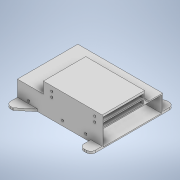
# Autodesk Inventor part: HardDriveHolder
Saved by Autodesk Inventor 2022 (Build 260153000, 153)
## iProperties
Created: 2021-08-26
Part Number: HardDriveHolder
Material: Generic
Document SubType Name: Modeling
Designer: anton
Density: 1 g/cm^3
Appearance: Default
Author: anton
Autodesk Inventor part; units mm, degrees
ref_plane "YZ Plane" through (0, 0, 0) normal (1, 0, 0) x (0, 1, 0)
ref_plane "XZ Plane" through (0, 0, 0) normal (0, 1, 0) x (-1, 0, 0)
ref_plane "XY Plane" through (0, 0, 0) normal (0, 0, 1) x (1, 0, 0)
sketch "Sketch1" plane through (0, 0, 0) normal (0, 1, 0) x (-1, 0, 0)
  line L0 (0, 0) -> (150, 0)
  line L1 (150, 0) -> (150, -107)
  line L2 (150, -107) -> (0, -107)
  line L3 (0, -107) -> (0, 0)
  dimension "d0" = 107
  dimension "d1" = 150
  constraints: 8 end point, 2 parallel, 1 horizontal, 1 perpendicular
  measures "d0" distance between parallel lines of L2 L0
  measures "d1" distance between parallel lines of L3 L1
extrude "Extrusion1" add sketch "Sketch1" along normal blind 32
sketch "Sketch3" plane through (0, 32, 0) normal (0, 1, 0) x (1, 0, 0)
  line L0 (-150, 0) -> (0, 0) projected
  line L1 (0, 0) -> (-104, 0)
  line L2 (-104, 0) -> (-104, 75)
  line L3 (-104, 75) -> (0, 75)
  line L4 (0, 75) -> (0, 0)
  dimension "d4" = 104
  dimension "d5" = 75
  constraints: 8 end point, 2 parallel, 1 horizontal, 1 perpendicular
  measures "d4" distance between parallel lines of L4 L2
  measures "d5" distance between parallel lines of L0 L3
extrude "Extrusion2" add sketch "Sketch3" along normal blind 20
sketch "Sketch4" plane through (0, 0, 0) normal (0, -1, 0) x (1, 0, 0)
  line L0 (0, 0) -> (0, -107) projected
  line L1 (0, 0) -> (-20, 0)
  line L2 (-20, 0) -> (-20, 12)
  line L3 (-12, 20) -> (-8, 20)
  line L4 (0, 12) -> (0, 0)
  line L5 (-150, -107) -> (-150, 0) projected
  line L6 (-150, 0) -> (-130, 0)
  line L7 (-138.364, 20) -> (-142, 20)
  line L8 (-150, 12) -> (-150, 0)
  line L9 (0, -107) -> (-150, -107) projected
  line L10 (-150, -107) -> (-130, -107)
  line L11 (-138.364, -127) -> (-142, -127)
  line L12 (-150, -119) -> (-150, -107)
  line L13 (0, -107) -> (-20, -107)
  line L14 (-20, -107) -> (-20, -119)
  line L15 (-12, -127) -> (-8, -127)
  line L16 (0, -119) -> (0, -107)
  arc A0 (0, 12) -> (-8, 20) centre (-8, 12) ccw
  arc A1 (-12, 20) -> (-20, 12) centre (-12, 12) ccw
  arc A2 (-8, -127) -> (0, -119) centre (-8, -119) ccw
  arc A3 (-20, -119) -> (-12, -127) centre (-12, -119) ccw
  arc A4 (-150, -119) -> (-142, -127) centre (-142, -119) ccw
  arc A5 (-142, 20) -> (-150, 12) centre (-142, 12) ccw
  line L17 (-150, 0) -> (0, 0) projected
  line L18 (-137.7212, -126.766) -> (-114.1649, -107)
  arc A6 (-138.364, -127) -> (-137.7212, -126.766) centre (-138.364, -126) ccw
  line L19 (-137.7212, 19.766) -> (-114.1649, 0)
  arc A7 (-137.7212, 19.766) -> (-138.364, 20) centre (-138.364, 19) ccw
  point P0 (-20, -127)
  dimension "d8" = 20
  dimension "d9" = 20
  dimension "d10" = 20
  dimension "d11" = 20
  dimension "d15" = 8
  dimension "d17" = 40
  dimension "d18" = 1
  dimension "d19" = 40
  dimension "d20" = 1
  constraints: 32 end point, 16 point on circle, 16 tangent, 8 centre point, 6 parallel, 5 equal radius, 5 point on line, 4 horizontal, 2 perpendicular
  measures "d8" distance between parallel lines of L2 L4
  measures "d9" distance between parallel lines of L1 L3
  measures "d10" distance between parallel lines of L15 L13
  measures "d11" distance between parallel lines of L14 L16
  measures "d15" radius of A0
  measures "d17" angle of L9 L18
  measures "d18" radius of A6
  measures "d19" angle of L17 L19
  measures "d20" radius of A7
extrude "Extrusion3" add sketch "Sketch4" against normal blind 4 contours L1 L2 A1 L3 A0 L4 | L16 A2 L15 A3 L14 L9 | L17 L6 L8 A5 L7 A7 L19 | L18 A6 L11 A4 L12 L9
sketch "Sketch5" plane through (0, 32, -75) normal (1, 0, 0) x (0, 0, -1)
  line L0 (-73, -2) -> (30, -2)
  line L1 (30, -2) -> (30, -30)
  line L2 (30, -30) -> (-73, -30)
  line L3 (-73, -30) -> (-73, -2)
  line L4 (-73, 16) -> (-2, 16)
  line L5 (-2, 16) -> (-2, 9)
  line L6 (-2, 9) -> (-73, 9)
  line L7 (-73, 9) -> (-73, 16)
  line L8 (-73, 7) -> (-2, 7)
  line L9 (-2, 7) -> (-2, 0)
  line L10 (-2, 0) -> (-73, 0)
  line L11 (-73, 0) -> (-73, 7)
  line L12 (-75, -28) -> (-75, 20) projected
  line L13 (-75, 20) -> (0, 20) projected
  line L14 (0, 0) -> (32, 0) projected
  point P0 (-75, -32)
  dimension "d23" = 7
  dimension "d24" = 7
  dimension "d25" = 28
  dimension "d26" = 71
  dimension "d27" = 71
  dimension "d28" = 2
  dimension "d29" = 2
  dimension "d31" = 2
  dimension "d32" = 2
  dimension "d33" = 103
  dimension "d34" = 2
  constraints: 24 end point, 6 parallel, 3 horizontal, 3 perpendicular, 1 point on line
  measures "d23" distance between parallel lines of L6 L4
  measures "d24" distance between parallel lines of L10 L8
  measures "d25" distance between parallel lines of L2 L0
  measures "d26" distance between parallel lines of L9 L11
  measures "d27" distance between parallel lines of L7 L5
  measures "d28" distance between parallel lines of L12 L7
  measures "d29" distance between parallel lines of L12 L11
  measures "d31" distance between parallel lines of L6 L8
  measures "d32" distance between parallel lines of L14 L0
  measures "d33" distance between parallel lines of L1 L3
  measures "d34" distance between parallel lines of L0 L10
extrude "Extrusion4" cut sketch "Sketch5" against normal blind 1000
fillet "Fillet1" radius 8 1 edges at (-52, 32, -75)
sketch "Sketch6" plane through (-104, 52, 0) normal (0, 0, 1) x (1, 0, 0)
  circle A0 centre (75, -43.5) radius 2
  circle A1 centre (34, -43.5) radius 2
  line L0 (104, -48) -> (104, 0) projected
  circle A2 centre (-26, -43.5) radius 2
  line L1 (-10.1649, -52) -> (84, -52) projected
  circle A3 centre (15, -8.5) radius 2
  circle A4 centre (91, -8.5) radius 2
  line L2 (0, -20) -> (0, 0) projected
  circle A5 centre (15, -17.5) radius 2
  circle A6 centre (91, -17.5) radius 2
  point P0 (104, -52)
  point P1 (104, -11)
  point P2 (104, -20)
  dimension "d38" = 29
  dimension "d39" = 41
  dimension "d40" = 0
  dimension "d42" = 0
  dimension "d43" = 60
  dimension "d44" = 4
  dimension "d45" = 4
  dimension "d46" = 4
  dimension "d47" = 8.5
  dimension "d48" = 0
  dimension "d49" = 76
  dimension "d50" = 15
  dimension "d51" = 4
  dimension "d52" = 4
  dimension "d53" = 2.5
  dimension "d54" = 4
  dimension "d55" = 4
  dimension "d56" = 2.5
  dimension "d57" = 2.5
  constraints: 7 centre point
  measures "d38" distance from line of L0 A0.centre
  measures "d39" distance of A1.centre A0.centre
  measures "d40" vertical distance of A0.centre A1.centre
  measures "d42" vertical distance of A2.centre A1.centre
  measures "d43" distance of A1.centre A2.centre
  measures "d44" diameter of A2
  measures "d45" diameter of A1
  measures "d46" diameter of A0
  measures "d47" distance from line of L1 A0.centre
  measures "d48" vertical distance of A4.centre A3.centre
  measures "d49" distance of A4.centre A3.centre
  measures "d50" distance from line of L2 A3.centre
  measures "d51" diameter of A3
  measures "d52" diameter of A4
  measures "d53" vertical distance of point (104, -11) A4.centre
  measures "d54" diameter of A6
  measures "d55" diameter of A5
  measures "d56" vertical distance of point (104, -20) A6.centre
  measures "d57" vertical distance of point (104, -20) A5.centre
extrude "Extrusion5" cut sketch "Sketch6" against normal blind 1000
body "Solid1"
